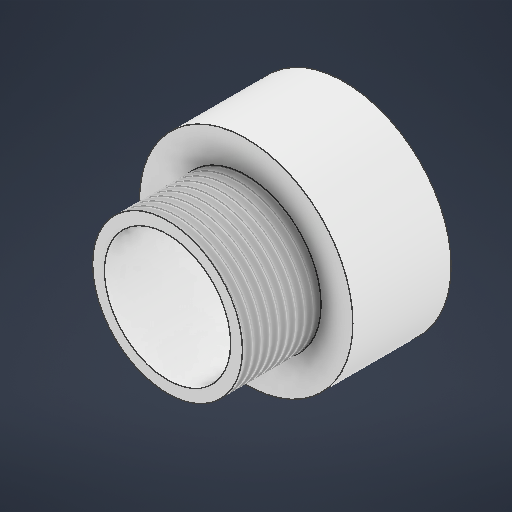
# Autodesk Inventor part: 1-1&2 FEMALE ADAPTER
Saved by Autodesk Inventor 2025.3 (Build 293356030, 356C)
## iProperties
Created: 2025-10-05
Part Number: 1-1&2 FEMALE ADAPTER
Material: Generic
Document SubType Name: Modeling
Designer: lstk1ng
Density: 1 g/cm^3
Appearance: Smooth - White
Author: lstk1ng
Autodesk Inventor part; units mm, degrees
ref_plane "YZ Plane" through (0, 0, 0) normal (1, 0, 0) x (0, 1, 0)
ref_plane "XZ Plane" through (0, 0, 0) normal (0, 1, 0) x (-1, 0, 0)
ref_plane "XY Plane" through (0, 0, 0) normal (0, 0, 1) x (1, 0, 0)
sketch "Sketch1" plane through (0, 0, 0) normal (0, 1, 0) x (-1, 0, 0)
  line L0 (0, 0) -> (-24.13, 0) construction
  line L1 (-24.13, 0) -> (-24.13, 22)
  line L2 (-19.05, 25) -> (-19.05, 45)
  line L3 (-24.13, 0) -> (-27.13, 0)
  line L4 (-27.13, 0) -> (-27.13, 25)
  line L5 (-27.13, 25) -> (-19.05, 25)
  line L6 (-27.13, 25) -> (-27.13, 25)
  line L7 (-27.13, 25) -> (-19.05, 25)
  line L8 (-19.05, 25) -> (-19.05, 25)
  line L9 (-19.05, 22) -> (-24.13, 22)
  line L10 (-16.05, 22) -> (-16.05, 45)
  line L11 (-19.05, 22) -> (-16.05, 22)
  line L12 (-16.05, 45) -> (-19.05, 45)
  line L13 (0, -9) -> (0, 54) projected
  dimension "d3" = 24.13
  dimension "d6" = 20
  dimension "d7" = 3
  dimension "d8" = 25
  constraints: 26 end point, 5 perpendicular, 4 horizontal, 1 point on line, 1 vertical
  measures "d3" distance of L0.start L0.end
  measures "d6" distance of L2.start L2.end
  measures "d7" distance of L0.end L3.end
  measures "d8" distance of L3.end L4.end
revolve "Revolution1" add sketch "Sketch1" angle 360 about axis through (0, 0, -10) along (0, 0, 1)
thread "Thread1" size "1 1/2" designation "1 1/2 - 11.5 NPT" standard "NPT for PVC Pipe and Fitting" length 26.04
body "Solid1"
